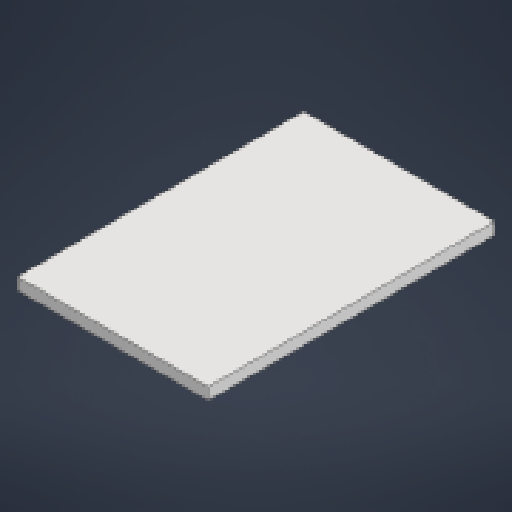
# Autodesk Inventor part: PCB_Housing_06_V4
Saved by Autodesk Inventor 2026.2 (Build 302298000, 298)
## iProperties
Created: 2026-03-17
Part Number: PCB_Housing_06_V4
Material: Generic
Document SubType Name: Modeling
Designer: vckot
Density: 1 g/cm^3
Appearance: Default
Author: vckot
Autodesk Inventor part; units mm, degrees
ref_plane "YZ Plane" through (0, 0, 0) normal (1, 0, 0) x (0, 1, 0)
ref_plane "XZ Plane" through (0, 0, 0) normal (0, 1, 0) x (-1, 0, 0)
ref_plane "XY Plane" through (0, 0, 0) normal (0, 0, 1) x (1, 0, 0)
sketch "Sketch1" plane through (0, 0, 0) normal (0, 1, 0) x (-1, 0, 0)
  line L0 (-40, 60) -> (40, 60)
  line L1 (40, 60) -> (40, -60)
  line L2 (40, -60) -> (-40, -60)
  line L3 (-40, -60) -> (-40, 60)
  line L4 (-40, 60) -> (40, -60) construction
  line L5 (40, 60) -> (-40, -60) construction
  point P0 (0, 0)
  dimension "d0" = 120
  dimension "d1" = 80
  constraints: 12 end point, 2 midpoint, 2 parallel, 1 horizontal, 1 perpendicular
  measures "d0" distance of L0.end L1.end
  measures "d1" distance of L0.start L0.end
extrude "Extrusion1" add sketch "Sketch1" along normal blind 5
sketch "Sketch2" plane through (0, 5, 0) normal (0, 1, 0) x (1, 0, 0)
  circle A0 centre (36.5, -56.5) radius 2.25 projected
  circle A1 centre (-36.5, 56.5) radius 2.25 projected
  point P0 (0, 0)
hole "Hole1" at (36.5, 5, 56.5) at (-36.5, 5, -56.5) direction (0, -1, 0) diameter 3.75 depth 8 tip angle 118 counterbore diameter 6 counterbore depth 3
sketch "Sketch3" plane through (0, 5, 0) normal (0, 1, 0) x (1, 0, 0)
  line L0 (22.241, -43.543499) -> (22.241, -20.556499)
  line L1 (8.779, -43.543499) -> (22.241, -43.543499)
  line L2 (8.779, -20.556499) -> (8.779, -43.543499)
  line L3 (8.779, -20.556499) -> (22.241, -20.556499)
  arc A0 (24.856832, 19.449996) -> (28.143167, 19.449996) centre (26.499999, 16.999996) ccw
  arc A1 (24.856832, 12.949996) -> (28.143167, 12.949996) centre (26.499999, 10.499996) ccw
  circle A2 centre (26.499999, 10.499996) radius 2.95
  circle A3 centre (26.499999, 16.999996) radius 2.95
  line L4 (28, 37.5) -> (-2, 37.5)
  line L5 (-2, 37.5) -> (-2, 51.5)
  line L6 (-2, 51.5) -> (28, 51.5)
  line L7 (28, 51.5) -> (28, 37.5)
  circle A4 centre (-7, 36) radius 1.1
  circle A5 centre (30, 36) radius 1.1
  circle A6 centre (30, 54) radius 1.1
  circle A7 centre (-7, 54) radius 1.1
  line L8 (31.5, 34.5) -> (31.5, 55.5)
  line L9 (31.5, 55.5) -> (-8.5, 55.5)
  line L10 (-8.5, 55.5) -> (-8.5, 34.5)
  line L11 (-8.5, 34.5) -> (31.5, 34.5)
  point P0 (0, 0)
  constraints: 2 centre point, 2 coincident, 2 concentric, 2 end point, 1 horizontal
extrude "Extrusion2" cut sketch "Sketch3" against normal through all contours L1 L2 L3 L0 | A3 A0 | A2 A1 | L4 L5 L6 L7 | A4 | A5 | A6 | A7 | L11 L10 L9 L8
thicken "Thicken1" operation add thickness 0.255 both sides no extend neighbours yes toward (0, 0, -1) faces at (18.166667, 1.666667, -55.5) (-8.5, 3.333333, -48.5) (31.5, 3.333333, -41.5) (4.833333, 1.666667, -34.5)
thicken "Thicken2" operation add thickness 0.25 both sides no extend neighbours yes toward (0.6830158, 0, -0.7304036) faces at (28.514896, 1.666667, -19.154687)
thicken "Thicken3" operation add thickness 0.25 both sides no extend neighbours yes toward (0.6830158, 0, -0.7304036) faces at (28.514896, 1.666667, -12.654687)
thicken "Thicken4" operation add thickness 0.25 both sides no extend neighbours yes toward (1, 0, 0) faces at (22.241, 3.333333, 35.881166) (13.266333, 1.666667, 20.556499) (8.779, 3.333333, 28.218832) (13.266333, 3.333333, 43.543499)
sketch "Sketch4" plane through (0, 5, 0) normal (0, 1, 0) x (1, 0, 0)
  line L0 (-10.777445, -22.968238) -> (9.753215, -22.968238) construction
  line L1 (9.753215, -22.968238) -> (9.753215, -46.641346) construction
  line L2 (9.753215, -46.641346) -> (-10.777444, -46.641347) construction
  line L3 (-10.777444, -46.641347) -> (-10.777445, -22.968238) construction
  line L4 (8.529, -20.306499) -> (22.491, -20.306499)
  spline S0 degree 2 poles (-5.844057, -23.793765) (-5.498028, -24.199113) (-5.112453, -25.385499) (-5.112453, -26.146763) knots 0 0 0 1 2 2 2
  spline S1 degree 2 poles (-5.112453, -26.146763) (-5.112453, -26.888254) (-5.488141, -28.08947) (-5.844057, -28.494819) knots 0 0 0 1 2 2 2
  spline S2 degree 2 poles (-5.844057, -28.494819) (-6.219746, -28.91994) (-7.213344, -29.325289) (-7.81148, -29.325289) knots 0 0 0 1 2 2 2
  spline S3 degree 2 poles (-7.81148, -29.325289) (-8.429389, -29.325289) (-9.418044, -28.90511) (-9.778903, -28.494819) knots 0 0 0 1 2 2 2
  spline S4 degree 2 poles (-9.778903, -28.494819) (-10.129876, -28.08947) (-10.505564, -26.898141) (-10.505564, -26.146763) knots 0 0 0 1 2 2 2
  spline S5 degree 2 poles (-10.505564, -26.146763) (-10.505565, -25.380556) (-10.124932, -24.213943) (-9.77396, -23.793765) knots 0 0 0 1 2 2 2
  spline S6 degree 2 poles (-9.77396, -23.793765) (-9.418044, -23.388417) (-8.424446, -22.968238) (-7.81148, -22.968238) knots 0 0 0 1 2 2 2
  spline S7 degree 2 poles (-7.81148, -22.968238) (-7.188628, -22.968238) (-6.190086, -23.403246) (-5.844057, -23.793765) knots 0 0 0 1 2 2 2
  spline S8 degree 2 poles (-5.957752, -26.146763) (-5.957752, -25.543684) (-6.219746, -24.609405) (-6.457023, -24.302922) knots 0 0 0 1 2 2 2
  spline S9 degree 2 poles (-6.457023, -24.302922) (-6.699244, -23.986553) (-7.381415, -23.670183) (-7.806537, -23.670183) knots 0 0 0 1 2 2 2
  spline S10 degree 2 poles (-7.806537, -23.670183) (-8.246488, -23.670183) (-8.908887, -23.976666) (-9.160994, -24.302922) knots 0 0 0 1 2 2 2
  spline S11 degree 2 poles (-9.160994, -24.302922) (-9.403214, -24.614348) (-9.660265, -25.553571) (-9.660265, -26.146763) knots 0 0 0 1 2 2 2
  spline S12 degree 2 poles (-9.660265, -26.146763) (-9.660265, -27.347979) (-8.651837, -28.623344) (-7.806537, -28.623344) knots 0 0 0 1 2 2 2
  spline S13 degree 2 poles (-7.806537, -28.623344) (-6.961237, -28.623344) (-5.957752, -27.347979) (-5.957752, -26.146763) knots 0 0 0 1 2 2 2
  line L5 (0.142248, -29.196763) -> (-0.767315, -29.196763)
  line L6 (-0.767315, -29.196763) -> (-3.466342, -23.93712)
  line L7 (-3.466342, -23.93712) -> (-3.466342, -29.196763)
  line L8 (-3.466342, -29.196763) -> (-4.222663, -29.196763)
  line L9 (-4.222663, -29.196763) -> (-4.222663, -23.096763)
  line L10 (-4.222663, -23.096763) -> (-3.07088, -23.096763)
  line L11 (-3.07088, -23.096763) -> (-0.614073, -27.926342)
  line L12 (-0.614073, -27.926342) -> (-0.614073, -23.096763)
  line L13 (-0.614073, -23.096763) -> (0.142248, -23.096763)
  line L14 (0.142248, -23.096763) -> (0.142248, -29.196763)
  spline S14 degree 2 poles (-5.844057, -33.837255) (-5.498028, -34.242603) (-5.112452, -35.428989) (-5.112452, -36.190253) knots 0 0 0 1 2 2 2
  spline S15 degree 2 poles (-5.112452, -36.190253) (-5.112452, -36.931744) (-5.488141, -38.13296) (-5.844057, -38.538308) knots 0 0 0 1 2 2 2
  spline S16 degree 2 poles (-5.844057, -38.538308) (-6.219746, -38.96343) (-7.213344, -39.368779) (-7.81148, -39.368779) knots 0 0 0 1 2 2 2
  spline S17 degree 2 poles (-7.81148, -39.368779) (-8.429389, -39.368779) (-9.418044, -38.9486) (-9.778903, -38.538309) knots 0 0 0 1 2 2 2
  spline S18 degree 2 poles (-9.778903, -38.538309) (-10.129875, -38.13296) (-10.505564, -36.941631) (-10.505564, -36.190253) knots 0 0 0 1 2 2 2
  spline S19 degree 2 poles (-10.505564, -36.190253) (-10.505564, -35.424046) (-10.124932, -34.257433) (-9.77396, -33.837255) knots 0 0 0 1 2 2 2
  spline S20 degree 2 poles (-9.77396, -33.837255) (-9.418044, -33.431906) (-8.424446, -33.011728) (-7.81148, -33.011728) knots 0 0 0 1 2 2 2
  spline S21 degree 2 poles (-7.81148, -33.011728) (-7.188627, -33.011728) (-6.190086, -33.446736) (-5.844057, -33.837255) knots 0 0 0 1 2 2 2
  spline S22 degree 2 poles (-5.957752, -36.190253) (-5.957752, -35.587174) (-6.219746, -34.652895) (-6.457023, -34.346412) knots 0 0 0 1 2 2 2
  spline S23 degree 2 poles (-6.457023, -34.346412) (-6.699243, -34.030043) (-7.381415, -33.713673) (-7.806537, -33.713673) knots 0 0 0 1 2 2 2
  spline S24 degree 2 poles (-7.806537, -33.713673) (-8.246488, -33.713673) (-8.908887, -34.020156) (-9.160994, -34.346412) knots 0 0 0 1 2 2 2
  spline S25 degree 2 poles (-9.160994, -34.346412) (-9.403214, -34.657838) (-9.660264, -35.59706) (-9.660264, -36.190253) knots 0 0 0 1 2 2 2
  spline S26 degree 2 poles (-9.660264, -36.190253) (-9.660264, -37.391469) (-8.651836, -38.666834) (-7.806537, -38.666834) knots 0 0 0 1 2 2 2
  spline S27 degree 2 poles (-7.806537, -38.666834) (-6.961237, -38.666834) (-5.957752, -37.391469) (-5.957752, -36.190253) knots 0 0 0 1 2 2 2
  line L15 (-0.574527, -33.861971) -> (-3.411966, -33.861971)
  line L16 (-3.411966, -33.861971) -> (-3.411966, -35.582231)
  line L17 (-3.411966, -35.582231) -> (-0.693165, -35.58223)
  line L18 (-0.693165, -35.58223) -> (-0.693165, -36.303948)
  line L19 (-0.693165, -36.303948) -> (-3.411966, -36.303949)
  line L20 (-3.411966, -36.303949) -> (-3.411966, -39.240253)
  line L21 (-3.411966, -39.240253) -> (-4.222663, -39.240253)
  line L22 (-4.222663, -39.240253) -> (-4.222663, -33.140253)
  line L23 (-4.222663, -33.140253) -> (-0.574527, -33.140253)
  line L24 (-0.574527, -33.140253) -> (-0.574527, -33.861971)
  line L25 (3.800271, -33.861971) -> (0.962831, -33.861971)
  line L26 (0.962831, -33.861971) -> (0.962831, -35.58223)
  line L27 (0.962831, -35.58223) -> (3.681632, -35.58223)
  line L28 (3.681632, -35.58223) -> (3.681632, -36.303948)
  line L29 (3.681632, -36.303948) -> (0.962831, -36.303948)
  line L30 (0.962831, -36.303948) -> (0.962832, -39.240253)
  line L31 (0.962832, -39.240253) -> (0.152135, -39.240253)
  line L32 (0.152135, -39.240253) -> (0.152134, -33.140253)
  line L33 (0.152134, -33.140253) -> (3.800271, -33.140253)
  line L34 (3.800271, -33.140253) -> (3.800271, -33.861971)
  point P0 (0, 0)
  dimension "d0" = 120
  dimension "d1" = 80
  constraints: 2 other
extrude "Extrusion3" cut sketch "Sketch4" against normal blind 2.5
body "Solid1"
